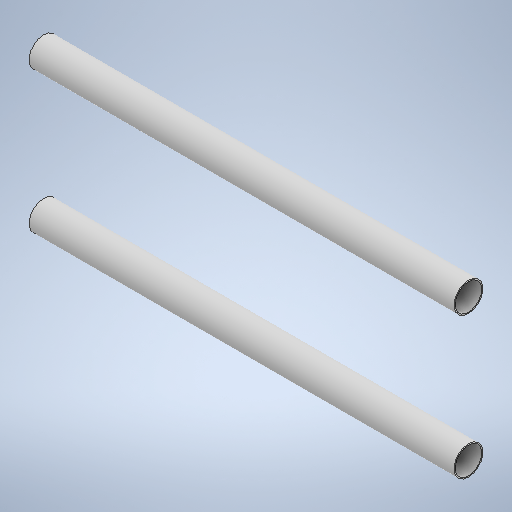
# Autodesk Inventor part: Trumpet
Saved by Autodesk Inventor 2025 (Build 290162010, 162A)
## iProperties
Created: 2025-01-16
Part Number: Trumpet
Material: Generic
Document SubType Name: Modeling
Designer: armenanzasn25
Density: 1 g/cm^3
Appearance: Default
Author: armenanzasn25
Autodesk Inventor part; units mm, degrees
ref_plane "YZ Plane" through (0, 0, 0) normal (1, 0, 0) x (0, 1, 0)
ref_plane "XZ Plane" through (0, 0, 0) normal (0, 1, 0) x (-1, 0, 0)
ref_plane "XY Plane" through (0, 0, 0) normal (0, 0, 1) x (1, 0, 0)
sketch "Sketch1" plane through (0, 0, 0) normal (1, 0, 0) x (0, 1, 0)
  circle A0 centre (33.8709, 0) radius 6.9215
  circle A1 centre (33.8709, 0) radius 6.3881
  circle A2 centre (-33.8709, 0) radius 6.9215
  circle A3 centre (-33.8709, 0) radius 6.3881
  point P0 (0, 0)
  dimension "d0" = 13.843
  dimension "d1" = 12.7762
  dimension "d2" = 67.7418
  dimension "d3" = 33.8709
  constraints: 4 centre point, 2 coincident, 2 equal radius, 2 horizontal alignment
  measures "d0" diameter of A0
  measures "d1" diameter of A1
  measures "d2" distance of A2.centre A0.centre
  measures "d3" distance of point (0, 0) A0.centre
extrude "Extrusion1" add sketch "Sketch1" along normal blind 203.2
equation "\"d0\" = TUBE_OUTER"
equation "\"d1\" = TUBE_INNER"
equation "\"d3\" = 0.5 * d2"
equation "\"TUBE_OUTER\" = 13.843"
equation "\"TUBE_INNER\" = 12.7762"
body "Solid1"
